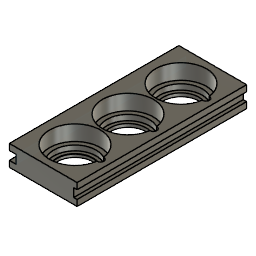
stop light (Autodesk Fusion 360 design; units mm, degrees)
Autodesk Fusion 360 part; units mm, degrees
sketch "Sketch1" plane through (0, 0, 0) normal (0, 0, 1) x (1, 0, 0)
  line L0 (0, 0) -> (40, 0)
  line L1 (40, 0) -> (40, 100)
  line L2 (40, 100) -> (0, 100)
  line L3 (0, 100) -> (0, 0)
  circle A0 centre (20, 50) radius 12.5
  circle A1 centre (20, 81.25) radius 12.5
  line L4 (5, 81.25, 3.25) -> (5, 66.25, 3.25)
  line L5 (5, 66.25, 3.25) -> (20, 66.25, 3.25)
  line L6 (35, 81.25, 3.25) -> (35, 96.25, 3.25)
  line L7 (35, 96.25, 3.25) -> (20, 96.25, 3.25)
  line L8 (35, 96.25, 3.25) -> (5, 96.25, 3.25)
  line L9 (5, 96.25, 3.25) -> (5, 66.25, 3.25)
  line L10 (5, 66.25, 3.25) -> (35, 66.25, 3.25)
  line L11 (35, 66.25, 3.25) -> (35, 96.25, 3.25)
  line L12 (5, 50, 3.25) -> (5, 65, 3.25)
  line L13 (5, 65, 3.25) -> (20, 65, 3.25)
  line L14 (35, 50, 3.25) -> (35, 35, 3.25)
  line L15 (35, 35, 3.25) -> (20, 35, 3.25)
  line L16 (35, 35, 3.25) -> (5, 35, 3.25)
  line L17 (5, 35, 3.25) -> (5, 65, 3.25)
  line L18 (5, 65, 3.25) -> (35, 65, 3.25)
  line L19 (35, 65, 3.25) -> (35, 35, 3.25)
  line L20 (5, 18.75, 3.25) -> (5, 3.75, 3.25)
  line L21 (5, 3.75, 3.25) -> (20, 3.75, 3.25)
  line L22 (35, 18.75, 3.25) -> (35, 33.75, 3.25)
  line L23 (35, 33.75, 3.25) -> (19.9836, 33.75, 3.25)
  line L24 (35, 33.75, 3.25) -> (5, 33.75, 3.25)
  line L25 (5, 33.75, 3.25) -> (5, 3.75, 3.25)
  line L26 (5, 3.75, 3.25) -> (35, 3.75, 3.25)
  line L27 (35, 3.75, 3.25) -> (35, 33.75, 3.25)
  circle A2 through (32.4836, 18.7208, 0.25) (13.7336, 29.5461, 0.25) (13.7336, 7.8955, 0.25)
  line L28 (5, 96.25, 3.25) -> (5, 100, 3.25) construction
  dimension "d1" = 40
  dimension "d2" = 100
  dimension "d11" = 25
  dimension "d15" = 25
  dimension "d55" = 25
  constraint horizontal L0
  constraint vertical L1
  constraint horizontal L2
  constraint vertical L3
  constraint coincident L0.start L3.end
  measures "d1" distance of L0.start L0.end
  measures "d2" distance of L0.start L2.end
  measures "d11" diameter of A0
  measures "d15" diameter of A1
extrude "Extrude1" add sketch "Sketch1" along normal blind 5 makes body 1
extrude "Extrude2" add sketch "Sketch1" against normal blind 2 separate body contours A0 | A1 makes body 2 at (19.2565, 46.7424, 0) makes body 3 at (19.0728, 79.6441, 0)
fillet "Fillet1" radius 2 4 faces at (19.0728, 79.6441, -2) (19.2565, 46.7424, -2) (19.2565, 46.7424, -2) (19.0728, 79.6441, -2) on bodies 2 3
extrude "Extrude3" cut 4 faces at (18.7213, 77.9918, -2) (17.2787, 53.4124, -2) (17.2787, 53.4124, -2) (18.7213, 77.9918, -2) along direction (0, 0, 1) blind 2 on bodies 2 3 bodies 2 3
extrude "Extrude7" cut sketch "Sketch1" along normal blind 10 contours L4 L5 L6 L7 L8 L9 L10 L11 | L12 L13 L14 L15 L16 L17 L18 L19 | L20 L21 L22 L23 L24 L25 L26 L27 in plane through (0, 0, 3.25) normal (0, 0, 1) bodies 1
extrude "Extrude8" add sketch "Sketch1" against normal blind 2 separate body contours A2 in plane through (0, 0, 0.25) normal (0, 0, 1) makes body 4
fillet "Fillet2" radius 2 1 faces at (16.5957, 18.0998, -1.75) on bodies 4
extrude "Extrude9" cut 1 faces at (23.1185, 23.5948, -1.75) along direction (0, 0, 1) blind 20 on bodies 4 bodies 1 4
extrude "Extrude10" cut 2 faces at (7.4992, 19.3439, 0.2497) (31.7315, 17.5781, 0.25) along direction (0, 0, 1) blind 8 on bodies 4 bodies 1
fillet "Fillet3" radius 15 4 edges at (5, 33.75, 4.125) (35, 33.75, 4.125) (5, 3.75, 4.125) (35, 3.75, 4.125) on bodies 1
fillet "Fillet4" radius 15 4 edges at (5, 65, 4.125) (35, 65, 4.125) (5, 35, 4.125) (35, 35, 4.125) on bodies 1
fillet "Fillet5" radius 15 4 edges at (5, 96.25, 4.125) (5, 66.25, 4.125) (35, 96.25, 4.125) (35, 66.25, 4.125) on bodies 1
extrude "Extrude11" add 1 faces at (1.6667, 49.999, 5) along direction (0, 0, 1) blind 7.25 on bodies 1 bodies 1
sketch "Sketch5" plane through (0, 0, 3.25) normal (0, 0, 1) x (1, 0, 0)
  line L0 (35, 81) -> (35, 85)
  circle A0 centre (35, 81) radius 2
  circle A1 centre (35, 50) radius 2
  circle A2 centre (35.0065, 18.7388) radius 2
  dimension "d85" = 4
  dimension "d86" = 4
  dimension "d87" = 4
  constraint vertical L0
  constraint coincident L0.start A0.centre
  measures "d85" diameter of A0
  measures "d86" diameter of A1
  measures "d87" diameter of A2
extrude "Extrude12" cut sketch "Sketch5" along normal blind 11 bodies 1
sketch "Sketch6" plane through (0, 0, 0) normal (-1, 0, 0) x (0, -1, 0)
  line L0 (-100, 0) -> (0, 0)
  line L1 (0, 0) -> (0, 12.25)
  line L2 (0, 12.25) -> (-100, 12.25)
  line L3 (-100, 12.25) -> (-100, 0)
  line L4 (0, 12.25) -> (0, 0) construction
  line L5 (0, 6.125) -> (0, 8.625) construction
  line L6 (0, 8.625) -> (-100, 8.625)
  line L7 (-100, 8.625) -> (-100, 3.625)
  line L8 (-100, 3.625) -> (0, 3.625)
  line L9 (0, 3.625) -> (0, 8.625)
  dimension "d90" = 2.5
  dimension "d91" = 100
  dimension "d92" = 5
  constraint coincident L1.end L2.start
  constraint coincident L0.end L1.start
  constraint midpoint L4 L5.start
  constraint perpendicular L0 L5
  constraint horizontal L6
  constraint vertical L7
  constraint horizontal L8
  constraint vertical L9
  measures "d90" distance of L5.start L5.end
  measures "d91" distance of L5.end L6.end
  measures "d92" distance of L5.end L8.end
extrude "Extrude13" cut sketch "Sketch6" against normal blind 4 contours L1 L3 L6 L7 L8 L9 bodies 1
sketch "Sketch7" plane through (4, 0, 0) normal (-1, 0, 0) x (0, -1, 0)
  line L0 (0, 3.625) -> (0, 8.625)
  line L1 (0, 8.625) -> (-100, 8.625)
  line L2 (-100, 8.625) -> (-100, 3.625)
  line L3 (-100, 3.625) -> (0, 3.625)
sketch "Sketch8" plane through (40, 0, 0) normal (1, 0, 0) x (0, 1, 0)
  line L0 (0, 0) -> (100, 0)
  line L1 (100, 0) -> (100, 12.25)
  line L2 (100, 12.25) -> (0, 12.25)
  line L3 (0, 12.25) -> (0, 0)
  line L4 (100, 6.125) -> (100, 8.625) construction
  line L5 (100, 8.625) -> (0, 8.625)
  line L6 (0, 8.625) -> (0, 3.625)
  line L7 (0, 3.625) -> (100, 3.625)
  line L8 (100, 3.625) -> (100, 8.625)
  dimension "d95" = 2.5
  dimension "d96" = 100
  dimension "d97" = 5
  constraint midpoint L1 L4.start
  constraint perpendicular L2 L4
  constraint horizontal L5
  constraint vertical L6
  constraint horizontal L7
  constraint vertical L8
  measures "d95" distance of L4.start L4.end
  measures "d96" distance of L4.end L5.end
  measures "d97" distance of L4.end L7.end
extrude "Extrude14" cut sketch "Sketch8" against normal blind 2 contours L1 L3 L5 L6 L7 L8 bodies 1
ref_plane "WorkPlane1" through (20, 18, 3) normal (0, 0, 1) x (1, 0, 0)
extrude "Extrude4" [suppressed]
extrude "Extrude5" [suppressed]
extrude "Extrude6" [suppressed]
